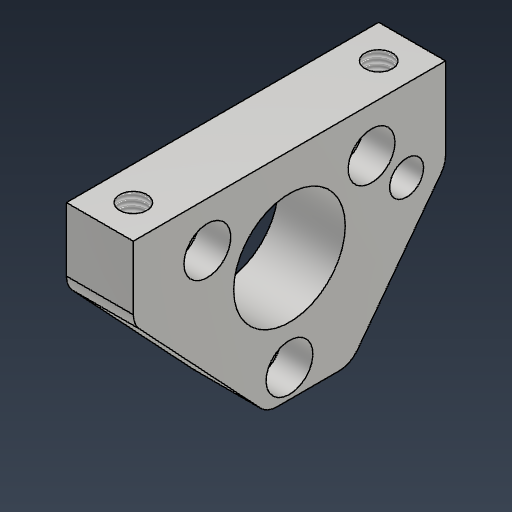
# Autodesk Inventor part: Motorhalter
Saved by Autodesk Inventor 2023.1 (Build 271208000, 208)
## iProperties
Part Number: Motorhalter
Material: Aluminium 6061
Document SubType Name: Modeling
Designer: rYan
Mass: 4.68408 g
Surface Area: 16.802 cm^2
Volume: 1.73484 cm^3
Density: 2.7 g/cm^3
Appearance: Aluminium - flach
Author: rYan
Autodesk Inventor part; units mm, degrees
ref_plane "YZ Plane" through (0, 0, 0) normal (1, 0, 0) x (0, 1, 0)
ref_plane "XZ Plane" through (0, 0, 0) normal (0, 1, 0) x (-1, 0, 0)
ref_plane "XY Plane" through (0, 0, 0) normal (0, 0, 1) x (1, 0, 0)
sketch "Skizze1" plane through (0, 0, 0) normal (1, 0, 0) x (0, 1, 0)
  arc A0 (-7.2187, 8.3) -> (7.2187, 8.3) centre (0, 0) ccw construction
  line L0 (14, 8.3) -> (-14, 8.3)
  line L1 (-14, 8.3) -> (-14, 1.8)
  line L2 (0, 12.16) -> (0, -14.86) projected
  circle A1 centre (0, 0) radius 5
  line L3 (14, 0.3) -> (14, 8.3)
  line L4 (-14, 1.8) -> (-2, -11)
  line L5 (-2, -11) -> (5.4841, -11)
  line L6 (5.4841, -11) -> (14, 0.3)
  circle A2 centre (10.504, 0.982) radius 1.525
  dimension "d0" = 22
  dimension "d2" = 10
  dimension "d19" = 8.3
  dimension "d39" = 14
  dimension "d50" = 3.05
  dimension "d57" = 10.504
  dimension "d61" = 2
  dimension "d62" = 6.5
  dimension "d63" = 8
  dimension "d86" = 10.5498
  dimension "d87" = 7.318
  dimension "d88" = 0.982
  constraints: 12 end point, 3 centre point, 2 coincident, 2 horizontal, 2 point on circle, 2 point on line, 2 tangent, 1 other
  measures "d0" diameter of A0
  measures "d2" diameter of A1
  measures "d19" distance from line of point (0, 0) L0
  measures "d39" distance between parallel lines of L1 L2
  measures "d50" diameter of A2
  measures "d57" horizontal distance of A2.centre point (0, 0)
  measures "d61" distance from line of L2 L4.end
  measures "d62" distance from line of L1.end L0
  measures "d63" distance of L3.start L0.start
  measures "d86" distance of A2.centre point (0, 0)
  measures "d87" distance from line of A2.centre L0
  measures "d88" vertical distance of point (0, 0) A2.centre
extrude "Extrusion1" add sketch "Skizze1" along normal mid plane 6 contours L3 L6 L5 L2 A1 L0 | L2 A1 L5 L4 L1 L0
sketch "Skizze2" plane through (3, 0, 0) normal (1, 0, 0) x (0, 0, -1)
  circle A0 centre (0, 0) radius 8.5 construction
  line L0 (0, 0) -> (8.5, 0) construction
  line L1 (-12.4, 0) -> (14.9, 0) projected
  dimension "d6" = 17
  constraints: 2 end point, 1 coincident, 1 horizontal alignment, 1 point on line, 2 other
hole "Bohrung1" at (3, 0, -8.5) direction (-1, 0, 0) diameter 2.1 end through all counterbore diameter 4.2 counterbore depth 2.8
pattern_circular "Runde Anordnung1" count 3 over 360 about axis through (0, 0, 0) along (1, 0, 0) of "Bohrung1"
sketch "Skizze3" plane through (-3, -14, 8.3) normal (0, 0, 1) x (1, 0, 0)
  line L0 (0, 0) -> (6, 0) projected
  line L1 (6, 28) -> (6, 0) projected
  line L2 (0, 0) -> (0, 28) projected
  line L3 (0, 0) -> (6, 0) construction
  line L4 (3, 0) -> (3, 24.0467) construction
  line L5 (6, 28) -> (0, 28) projected
  line L6 (-1.2, 14) -> (7.2, 14) projected
  point P0 (3, 14)
  point P1 (3, 3)
  point P2 (3, 25)
  dimension "d44" = 11
  constraints: 2 end point, 2 point on line, 1 midpoint, 1 symmetric about line
  measures "d44" distance of point (3, 3) point (3, 14)
hole "Bohrung2" at (0, -11, 8.3) at (0, 11, 8.3) direction (0, 0, -1) diameter 2.459 depth 6 tip angle 118 thread size "M3x0.5" class "6H" standard "ISO Metric profile"
fillet "Rundung2" radius 2 4 edges at (0, -2, -11) (0, 5.4841, -11) (0, -14, 1.8) (0, 14, 0.3)
sketch "Skizze7" plane through (-3, -14, 8.3) normal (0, 0, 1) x (1, 0, 0)
  line L0 (3, 33.6) -> (3, -5.6) construction
  line L1 (-1.2, 14) -> (7.2, 14) construction
  point P0 (3, 14)
  point P1 (3, 10)
  point P2 (3, 18)
  dimension "d78" = 8
  constraints: 2 point on line, 1 symmetric about line
  measures "d78" distance of point (3, 18) point (3, 10)
hole "Bohrung4" [suppressed]
sketch "Skizze6" plane through (3, 0, 0) normal (1, 0, 0) x (0, 0, -1)
  circle A0 centre (0.5, -7.5) radius 1.5
  circle A1 centre (0.5, -7.5) radius 3 construction
  circle A2 centre (-0.982, 10.504) radius 1.525 construction
  circle A3 centre (-0.982, 10.504) radius 2.75 construction
  circle A4 centre (3, 7.5) radius 3 construction
  circle A5 centre (3, 7.5) radius 1.5
  line L0 (-1.223, -13.4591) -> (10.3679, -2.5926) construction
  line L1 (10.2037, 6.0842) -> (0.2345, 13.5972) construction
  circle A6 centre (-4.25, -7.3612) radius 2.1 construction
  circle A7 centre (0, 0) radius 5 construction
  dimension "d64" = 3
  dimension "d65" = 6
  dimension "d66" = 5.5
  dimension "d67" = 6
  dimension "d68" = 3
  dimension "d69" = 1.152
  dimension "d70" = 1.963
  dimension "d71" = 7.5
  dimension "d72" = 0.5
  dimension "d73" = 7.5
  dimension "d74" = 3
  dimension "d75" = 1.0167
  constraints: 5 centre point, 3 coincident
  measures "d64" diameter of A0
  measures "d65" diameter of A1
  measures "d66" diameter of A3
  measures "d67" diameter of A4
  measures "d68" diameter of A5
  measures "d71" vertical distance of A0.centre point (0, 0)
  measures "d72" horizontal distance of point (0, 0) A0.centre
  measures "d73" vertical distance of point (0, 0) A4.centre
  measures "d74" horizontal distance of point (0, 0) A4.centre
extrude "Fräshalterung Schrauben" [suppressed]
